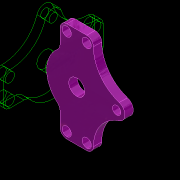
# Autodesk Inventor part: ShufflerPodEndPlate
Saved by Autodesk Inventor 2022 (Build 260153000, 153)
## iProperties
Created: 2022-03-06
Part Number: ShufflerPodEndPlate
Material: Custom TPU
Document SubType Name: Modeling
Designer: tandu
Density: 1.21 g/cm^3
Appearance: Smooth - Purple
Author: tandu
Autodesk Inventor part; units mm, degrees
ref_plane "YZ Plane" through (0, 0, 0) normal (1, 0, 0) x (0, 1, 0)
ref_plane "XZ Plane" through (0, 0, 0) normal (0, 1, 0) x (-1, 0, 0)
ref_plane "XY Plane" through (0, 0, 0) normal (0, 0, 1) x (1, 0, 0)
sketch "Sketch1" plane through (0, 0, 0) normal (0, 0, 1) x (1, 0, 0)
  circle A0 centre (-1.4287, 16.51) radius 2.54 projected
  circle A1 centre (-9.0487, 16.51) radius 2.54 projected
  circle A2 centre (-9.0487, -16.51) radius 2.54 projected
  circle A3 centre (-1.4287, -16.51) radius 2.54 projected
  circle A4 centre (10.0012, 0) radius 1.5875 projected
  circle A5 centre (-5.2387, 0) radius 3.048 projected
  arc A6 (-9.0487, -19.05) -> (-11.5887, -16.51) centre (-9.0487, -16.51) ccw projected
  line L0 (-9.0487, -19.05) -> (-1.4287, -19.05) projected
  arc A7 (1.1112, -16.51) -> (-1.4287, -19.05) centre (-1.4287, -16.51) ccw projected
  arc A8 (9.5738, -3.175) -> (1.1112, -16.51) centre (15.8489, -16.51) ccw construction
  arc A9 (9.5738, -3.175) -> (11.5887, 0) centre (8.0798, 0) ccw construction
  circle A10 centre (10.0012, 0) radius 1.5875 projected
  arc A11 (11.5887, 0) -> (9.5738, 3.175) centre (8.0798, 0) ccw construction
  arc A12 (1.1112, 16.51) -> (9.5738, 3.175) centre (15.8489, 16.51) ccw construction
  arc A13 (-1.4287, 19.05) -> (1.1112, 16.51) centre (-1.4287, 16.51) ccw projected
  line L1 (-1.4287, 19.05) -> (-9.0487, 19.05) projected
  arc A14 (-11.5887, 16.51) -> (-9.0487, 19.05) centre (-9.0487, 16.51) ccw projected
  line L2 (-11.5887, 16.51) -> (-11.5887, 11.123) projected
  arc A15 (-12.6986, 8.7114) -> (-11.5887, 11.123) centre (-14.7637, 11.123) ccw projected
  arc A16 (-12.6986, 8.7114) -> (-12.6986, -8.7114) centre (-5.2387, 0) ccw projected
  arc A17 (-11.5887, -11.123) -> (-12.6986, -8.7114) centre (-14.7637, -11.123) ccw projected
  line L3 (-11.5887, -11.123) -> (-11.5887, -16.51) projected
  circle A18 centre (-1.4287, 16.51) radius 1.7526
  circle A19 centre (-9.0487, 16.51) radius 1.7526
  circle A20 centre (-9.0487, -16.51) radius 1.7526
  circle A21 centre (-1.4287, -16.51) radius 1.7526
  circle A22 centre (10.0012, 0) radius 3.175
  arc A23 (1.1112, 16.51) -> (10.9657, 3.025) centre (15.2651, 16.51) ccw
  arc A24 (10.9657, -3.025) -> (1.1112, -16.51) centre (15.2651, -16.51) ccw
  point P0 (0, 0)
  dimension "d0" = 3.5052
  dimension "d1" = 1.5875
  constraints: 7 centre point, 6 point on circle, 4 coincident, 4 tangent, 3 equal radius, 2 horizontal alignment
  measures "d0" diameter of A18
extrude "Extrusion1" add sketch "Sketch1" along normal blind 3.175
body "Solid1"
